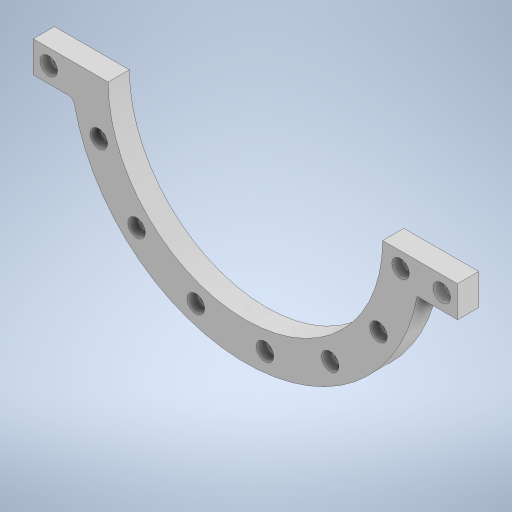
# Autodesk Inventor part: Постель 201 зад
Saved by Autodesk Inventor 2024.2 (Build 282272000, 272)
## iProperties
Created: 2024-04-28
Part Number: Постель 201 зад
Material: Generic
Document SubType Name: Modeling
Designer: admin
Density: 1 g/cm^3
Appearance: Default
Author: pokla
Autodesk Inventor part; units mm, degrees
ref_plane "YZ Plane" through (0, 0, 0) normal (1, 0, 0) x (0, 1, 0)
ref_plane "XZ Plane" through (0, 0, 0) normal (0, 1, 0) x (-1, 0, 0)
ref_plane "XY Plane" through (0, 0, 0) normal (0, 0, 1) x (1, 0, 0)
sketch "Sketch1" plane through (0, 0, 0) normal (0, 0, 1) x (1, 0, 0)
  circle A0 centre (0, 0) radius 250 construction
  line L0 (0, 250) -> (0, 280) construction
  line L1 (0, 250) -> (0, 220) construction
  circle A1 centre (0, 0) radius 220
  circle A2 centre (0, 0) radius 280
  line L2 (-220, 0) -> (-220, 80)
  line L3 (-220, 80) -> (-280, 80)
  line L4 (-280, 80) -> (-280, 0)
  line L5 (220, 0) -> (220, 80)
  line L6 (220, 80) -> (280, 80)
  line L7 (280, 80) -> (280, 0)
  line L8 (-220, 0) -> (-280, 0)
  line L9 (-280, 0) -> (-340, 0)
  line L10 (-340, 0) -> (-340, -50)
  line L11 (-340, -50) -> (-275.4995, -50)
  line L12 (220, 0) -> (280, 0)
  line L13 (280, 0) -> (340, 0)
  line L14 (340, 0) -> (340, -50)
  line L15 (340, -50) -> (275.4995, -50)
  dimension "d13" = 500
  dimension "d26" = 80
  dimension "d36" = 60
  dimension "d40" = 60
  dimension "d41" = 50
  constraints: 32 end point, 8 point on circle, 7 perpendicular, 4 equal length, 4 horizontal, 4 tangent, 4 vertical, 3 coincident, 2 centre point, 1 line through centre, 1 point on line, 1 vertical alignment, 2 other
  measures "d26" distance of L2.start L2.end
  measures "d36" distance of L1.end L0.end
  measures "d40" distance of L4.end L9.end
  measures "d41" distance of L9.end L10.end
extrude "Extrusion1" add sketch "Sketch1" against normal blind 34 contours L12 A2 L8 A1 | L13 L14 L15 A2 | A2 L11 L10 L9
sketch "Sketch4" plane through (0, 0, 0) normal (0, 0, 1) x (1, 0, 0)
  line L0 (0, 0) -> (31.5497, -248.0012) construction
  line L1 (0, 0) -> (0, -276.8337) construction
  dimension "d27" = 250
  dimension "d35" = 7.25
  constraints: 4 end point, 1 coincident, 1 vertical
  measures "d27" distance of L0.end L0.start
  measures "d35" angle of L1 L0
sketch "Sketch7" plane through (0, 0, 0) normal (0, 0, 1) x (1, 0, 0)
  line L0 (-340, -50) -> (-340, 0) construction
  line L1 (-340, -25) -> (340, -25) construction
  line L2 (340, 0) -> (340, -50) construction
  point P0 (0, 0)
  point P1 (-315, -25)
  dimension "d42" = 25
  constraints: 2 end point, 2 midpoint, 1 point on line
  measures "d42" distance from line of point (-315, -25) L0
fillet "Fillet1" radius 10 1 edges at (-275.4995, -50, -17)
hole "Hole1" at (-315, -25, 0) direction (0, 0, -1) diameter 18 end through all counterbore diameter 28 counterbore depth 15
hole "Hole2" at (31.5497, -248.0012, 0) direction (0, 0, -1) diameter 18 end through all counterbore diameter 28 counterbore depth 15
pattern_circular "Circular Pattern4" count 8 over 180 about axis through (0, 0, -10) along (0, 0, -1) of "Hole2" both ways yes
mirror "Mirror1" about plane through (0, 0, 0) normal (1, 0, 0) of "Hole1"
equation "\"d13\" = Шпил_пласт_КОРМА_диам_центров"
equation "\"d40\" = d36"
equation "\"d27\" = 0.5 * Шпил_пласт_КОРМА_диам_центров"
equation "\"Шпил_пласт_КОРМА_диам_центров\" = 500"
body "Solid1"
